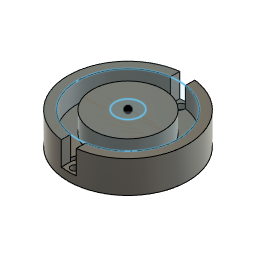
Solenoid Tool Path (Autodesk Fusion 360 design; units mm, degrees)
Autodesk Fusion 360 part; units mm, degrees
note: some values were not read from the file. Set by a fixed rule: which sketch regions a step uses.
sketch "Sketch1" plane through (0, 0, 0) normal (0, 1, 0) x (1, 0, 0)
  circle A0 centre (0, 0) radius 50.5
  dimension "d1" = 101
  constraint coincident A0.centre origin
  measures "d1" diameter of A0
extrude "Extrude1" add sketch "Sketch1" along normal blind 27
sketch "Sketch2" plane through (0, 27, 0) normal (0, 1, 0) x (-1, 0, 0)
  circle A0 centre (0, 0) radius 50.5
  circle A1 centre (0, 0) radius 42.7
  circle A2 centre (0, 0) radius 30
  dimension "d4" = 85.4
  dimension "d5" = 60
  constraint concentric A0 A1
  constraint concentric A1 A2
  measures "d4" diameter of A1
  measures "d5" diameter of A2
extrude "Extrude2" cut sketch "Sketch2" against normal blind 17 contours A1
sketch "Sketch3" plane through (0, 27, 0) normal (0, 1, 0) x (-1, 0, 0)
  circle A0 centre (0, 0) radius 30
  line L0 (-21.2901, 0) -> (20, 0)
  line L1 (6.35, -35) -> (-6.35, -35)
  line L2 (-6.35, -35) -> (-6.35, -60)
  line L3 (-6.35, -60) -> (6.35, -60)
  line L4 (6.35, -60) -> (6.35, -35)
  line L5 (12.7006, 0) -> (-15, 0)
  line L6 (6.35, 60) -> (6.35, 35)
  line L7 (-6.35, 60) -> (6.35, 60)
  line L8 (-6.35, 35) -> (-6.35, 60)
  line L9 (6.35, 35) -> (-6.35, 35)
  line L10 (0, 15) -> (0, 0)
  dimension "d8" = 12.7
  dimension "d9" = 6.35
  constraint horizontal L0
  constraint horizontal L1
  constraint vertical L2
  constraint horizontal L3
  constraint vertical L4
  constraint coincident L0 L5.start
  constraint coincident L0 L5.end
  constraint symmetric L1.start L5 L6.end
  constraint symmetric L1.end L5 L8.start
  constraint symmetric L2.end L5 L7.start
  constraint symmetric L3.end L5 L6.start
  constraint perpendicular L5 L10
  constraint coincident A0.centre L10.end
  measures "d8" distance of L2.end L3.end
  measures "d9" distance of L4 L10
extrude "Extrude3" cut sketch "Sketch3" against normal blind 17 contours L1 L2 L3 L4 | L6 L7 L8 L9
sketch "Sketch4" plane through (0, 10, 0) normal (0, 1, 0) x (-1, 0, 0)
  arc A0 (-6.35, 42.2252) -> (-6.35, -42.2252) centre (0, 0) ccw
  line L0 (-6.35, -42.2252) -> (-6.35, -50.0992)
  arc A1 (-6.35, -50.0992) -> (6.35, -50.0992) centre (0, 0) ccw
  line L1 (6.35, -50.0992) -> (6.35, -42.2252)
  arc A2 (6.35, -42.2252) -> (6.35, 42.2252) centre (0, 0) ccw
  line L2 (6.35, 42.2252) -> (6.35, 50.0992)
  arc A3 (6.35, 50.0992) -> (-6.35, 50.0992) centre (0, 0) ccw
  line L3 (-6.35, 50.0992) -> (-6.35, 42.2252)
  circle A4 centre (0, 0) radius 30
  line L4 (0, 0) -> (0, 65)
  line L5 (0, 65) -> (0, -75)
  circle A5 centre (0, -45.0375) radius 3.3
  line L6 (18, 0) -> (-17, 0)
  circle A6 centre (0, 45.0375) radius 3.3
  dimension "d12" = 6.6
  dimension "d17" = 45.0375
  dimension "d18" = 45.0375
  constraint coincident A0.centre A1.centre
  constraint parallel L2 L4
  constraint parallel L4 L5
  constraint coincident L5 A5.centre
  constraint horizontal L6
  constraint symmetric A5 L6 A6
  measures "d12" diameter of A5
  measures "d17" distance of A0.centre A5.centre
  measures "d18" distance of A0.centre A6.centre
extrude "Extrude4" cut sketch "Sketch4" against normal up to surface (10 mm away) contours L4 L5 A6 | L4 L5 A6 | L5 A5 | L5 A5
sketch "Sketch5" plane through (0, 10, 0) normal (0, 1, 0) x (-1, 0, 0)
  circle A0 centre (0, -45.0375) radius 3.3
  circle A1 centre (0, 45.0375) radius 3.3
  arc A2 (-6.35, 42.2252) -> (-6.35, -42.2252) centre (0, 0) ccw
  line L0 (-6.35, -42.2252) -> (-6.35, -50.0992)
  arc A3 (-6.35, -50.0992) -> (6.35, -50.0992) centre (0, 0) ccw
  line L1 (6.35, -50.0992) -> (6.35, -42.2252)
  arc A4 (6.35, -42.2252) -> (6.35, 42.2252) centre (0, 0) ccw
  line L2 (6.35, 42.2252) -> (6.35, 50.0992)
  arc A5 (6.35, 50.0992) -> (-6.35, 50.0992) centre (0, 0) ccw
  line L3 (-6.35, 50.0992) -> (-6.35, 42.2252)
  circle A6 centre (0, 0) radius 30
  circle A7 centre (0, -42.2252) radius 6.35
  line L4 (12.9557, 0.0186) -> (-15, 0.0186)
  circle A8 centre (0, 42.2624) radius 6.35
  constraint coincident A2.end A7
  constraint tangent L0 A7
  constraint coincident L1.end A7
  constraint horizontal L4
  constraint symmetric A7 L4 A8
extrude "Extrude5" cut sketch "Sketch5" against normal blind 3 contours L2 A5 L3 A8 | L2 A8 | L0 A3 L1 A7 | A7
ref_plane "WorkPlane1" through (0, 27.508, 0) normal (0, 1, 0) x (1, 0, 0)
sketch "Sketch6" plane through (0, 27.508, 0) normal (0, 1, 0) x (1, 0, 0)
  circle A0 centre (0, 0) radius 10.6711
  constraint coincident A0.centre origin
sketch "Sketch7" plane through (0, 27, 0) normal (0, 1, 0) x (-1, 0, 0)
  line L0 (6.35, 50.0992) -> (6.35, 42.2252)
  arc A0 (6.35, -42.2252) -> (6.35, 42.2252) centre (0, 0) ccw
  line L1 (6.35, -42.2252) -> (6.35, -50.0992)
  arc A1 (6.35, -50.0992) -> (6.35, 50.0992) centre (0, 0) ccw
  circle A2 centre (0, 0) radius 42.7
  constraint coincident A0.centre A1.centre
equation "d4 = 60 mm + 1 in"
equation "d9 = 0.5 in / 2"
equation "d17 = 1.8125 in - 1 mm"
equation "d18 = d17"
